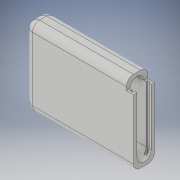
# Autodesk Inventor part: Marcus' Case
Saved by Autodesk Inventor 2018 (Build 220112000, 112)
## iProperties
Created: 2019-09-03
Part Number: Marcus' Case
Material: Generic
Document SubType Name: Modeling
Designer: 871357
Density: 1 g/cm^3
Appearance: Default
Author: 871357
Autodesk Inventor part; units mm, degrees
ref_plane "YZ Plane" through (0, 0, 0) normal (1, 0, 0) x (0, 1, 0)
ref_plane "XZ Plane" through (0, 0, 0) normal (0, 1, 0) x (-1, 0, 0)
ref_plane "XY Plane" through (0, 0, 0) normal (0, 0, 1) x (1, 0, 0)
sketch "Sketch1" plane through (0, 0, 0) normal (0, 0, 1) x (1, 0, 0)
  line L0 (0, 0) -> (-87.63, 0)
  line L1 (-87.63, 0) -> (-87.63, 63.5)
  line L2 (-87.63, 63.5) -> (0, 63.5)
  line L3 (0, 63.5) -> (0, 0)
  dimension "d0" = 87.63
  dimension "d1" = 63.5
  constraints: 8 end point, 2 parallel, 1 horizontal, 1 perpendicular
  measures "d0" distance of L1.end L2.end
  measures "d1" distance of L0.end L1.end
sketch "Sketch2" plane through (0, 0, 0) normal (0, 0, 1) x (1, 0, 0)
  line L0 (0, -3.175) -> (-90.805, -3.175)
  line L1 (-90.805, -3.175) -> (-90.805, 66.675)
  line L2 (-90.805, 66.675) -> (0, 66.675)
  line L3 (0, 66.675) -> (0, -3.175)
  line L4 (-87.63, 63.5) -> (0, 63.5) projected
  point P0 (0, 0)
  dimension "d2" = 3.175
  dimension "d3" = 3.175
  dimension "d4" = 66.675
  dimension "d6" = 0
  constraints: 8 end point, 2 parallel, 1 horizontal, 1 perpendicular
  measures "d2" distance between parallel lines of L4 L2
  measures "d3" distance from line of L4.start L1
  measures "d4" distance between parallel lines of L4 L0
  measures "d6" distance from line of L4.end L3
extrude "Extrusion1" add sketch "Sketch2" along normal mid plane 19.05
extrude "Extrusion2" cut sketch "Sketch1" along normal mid plane 12.7
fillet "Fillet1" radius 6.35 16 edges at (-43.815, 63.5, 6.35) (-43.815, 63.5, -6.35) (-43.815, 0, -6.35) (-45.4025, -3.175, 9.525) (-43.815, 0, 6.35) (-45.4025, -3.175, -9.525) (-90.805, 31.75, -9.525) (-90.805, -3.175, 0) (-90.805, 31.75, 9.525) (-90.805, 66.675, 0) (-45.4025, 66.675, -9.525) (-45.4025, 66.675, 9.525) (-87.63, 31.75, 6.35) (-87.63, 31.75, -6.35) (-87.63, 63.5, 0) (-87.63, 0, 0)
sketch "Sketch3" plane through (0, 3.175, -9.525) normal (1, 0, 0) x (0, 0, -1)
  line L0 (-3.175, 53.975) -> (-3.175, 3.175) projected
  arc A0 (-15.875, 3.175) -> (-3.175, 3.175) centre (-9.525, 3.175) ccw projected
  line L1 (-15.875, 3.175) -> (-15.875, 53.975) projected
  arc A1 (-3.175, 53.975) -> (-15.875, 53.975) centre (-9.525, 53.975) ccw construction
  arc A2 (-19.05, 0) -> (-12.7, -6.35) centre (-12.7, 0) ccw projected
  line L2 (-6.35, -6.35) -> (-12.7, -6.35) projected
  arc A3 (-6.35, -6.35) -> (0, 0) centre (-6.35, 0) ccw projected
  line L3 (0, 57.15) -> (0, 0) construction
  arc A4 (0, 57.15) -> (-6.35, 63.5) centre (-6.35, 57.15) ccw construction
  line L4 (-12.7, 63.5) -> (-6.35, 63.5) construction
  arc A5 (-12.7, 63.5) -> (-19.05, 57.15) centre (-12.7, 57.15) ccw construction
  line L5 (-19.05, 0) -> (-19.05, 57.15) construction
  line L6 (-19.05, 0) -> (-19.05, 53.975)
  line L7 (-19.05, 0) -> (-19.05, 57.15) construction
  line L8 (0, 0) -> (-6.35, 0) construction
  line L9 (0, 0) -> (0, 53.975)
  line L10 (0, 57.15) -> (0, 0) construction
  line L11 (-19.05, 53.975) -> (-15.875, 53.975)
  line L12 (0, 53.975) -> (-3.175, 53.975)
  point P0 (-9.525, -3.175)
  constraints: 8 end point, 2 point on line, 1 horizontal, 1 perpendicular
extrude "Extrusion3" add sketch "Sketch3" along normal blind 6.35
sketch "Sketch4" plane through (0, 57.15, 9.525) normal (0, 1, 0) x (1, 0, 0)
  line L0 (6.35, 15.875) -> (-81.28, 15.875) construction
  line L1 (4.445, 15.875) -> (1.905, 15.875) construction
  line L2 (1.905, 15.875) -> (1.905, 17.4625)
  line L3 (1.905, 17.4625) -> (4.445, 17.4625)
  line L4 (4.445, 17.4625) -> (4.445, 15.875)
  line L5 (6.35, 19.05) -> (6.35, 15.875) construction
  line L6 (-3.9045, 9.525) -> (6.35, 9.525) construction
  line L7 (1.905, 3.175) -> (1.905, 1.5875)
  line L8 (1.905, 1.5875) -> (4.445, 1.5875)
  line L9 (4.445, 1.5875) -> (4.445, 3.175)
  line L10 (0, 3.175) -> (6.35, 3.175) construction
  line L11 (1.905, 15.875) -> (1.905, 13.9011)
  line L12 (1.905, 13.9011) -> (4.445, 13.9011)
  line L13 (4.445, 13.9011) -> (4.445, 15.875)
  line L14 (4.445, 3.175) -> (4.445, 4.5966)
  line L15 (4.445, 4.5966) -> (1.905, 4.5966)
  line L16 (1.905, 4.5966) -> (1.905, 3.175)
  point P0 (0, 9.525)
  dimension "d14" = 2.54
  dimension "d15" = 1.5875
  dimension "d16" = 1.905
  constraints: 28 end point, 4 perpendicular, 4 symmetric about line, 2 horizontal, 2 parallel, 2 vertical, 1 collinear, 1 point on line
  measures "d14" distance of L2.end L3.end
  measures "d15" distance of L1.end L2.end
  measures "d16" distance between parallel lines of L4 L5
extrude "Extrusion4" cut sketch "Sketch4" against normal blind 55.88
body "Solid1"
